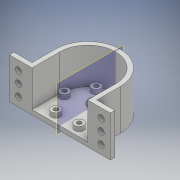
# Autodesk Inventor part: Mount for run motor
Saved by Autodesk Inventor 2018 (Build 220112000, 112)
## iProperties
Created: 2020-02-06
Part Number: Mount for run motor
Material: Типовые
Document SubType Name: Modeling
Designer: cosko
Density: 1 g/cm^3
Appearance: По умолчанию
Author: cosko
Autodesk Inventor part; units mm, degrees
ref_plane "YZ Plane" through (0, 0, 0) normal (1, 0, 0) x (0, 1, 0)
ref_plane "XZ Plane" through (0, 0, 0) normal (0, 1, 0) x (-1, 0, 0)
ref_plane "XY Plane" through (0, 0, 0) normal (0, 0, 1) x (1, 0, 0)
sketch "Эскиз1" plane through (0, 0, 0) normal (0, 0, 1) x (1, 0, 0)
  line L0 (0, 0) -> (0, 37) construction
  circle A0 centre (0, 18.5) radius 18.5 construction
  arc A1 (10.9545, 0) -> (-10.9545, 0) centre (0, 18.5) ccw construction
  line L1 (21.5, 18.5) -> (21.5, 0) construction
  line L2 (-21.5, 18.5) -> (-21.5, 0) construction
  line L3 (-21.5, 0) -> (21.5, 0) construction
  arc A2 (21.5, 18.5) -> (-21.5, 18.5) centre (0, 18.5) ccw construction
  arc A3 (21.5, 18.5) -> (-21.5, 18.5) centre (0, 18.5) ccw
  arc A4 (18.5, 18.5) -> (-18.5, 18.5) centre (0, 18.5) ccw
  line L4 (21.5, 0) -> (33.5, 0) construction
  line L5 (-21.5, 0) -> (-33.5, 0) construction
  line L6 (33.5, 0) -> (33.5, 3) construction
  line L7 (33.5, 3) -> (21.5, 3) construction
  line L8 (21.5, 3) -> (21.5, 18.5) construction
  line L9 (-33.5, 0) -> (-33.5, 3) construction
  line L10 (-33.5, 3) -> (-21.5, 3) construction
  line L11 (-21.5, 18.5) -> (-21.5, 3)
  line L12 (-21.5, 3) -> (-33.5, 3)
  line L13 (-33.5, 3) -> (-33.5, 0)
  line L14 (-33.5, 0) -> (-18.5, 0)
  line L15 (-18.5, 0) -> (-18.5, 18.5)
  line L16 (18.5, 18.5) -> (18.5, 0)
  line L17 (18.5, 0) -> (33.5, 0)
  line L18 (33.5, 0) -> (33.5, 3)
  line L19 (33.5, 3) -> (21.5, 3)
  line L20 (21.5, 3) -> (21.5, 18.5)
  dimension "d0" = 37
  dimension "d1" = 3
  dimension "d2" = 12
  dimension "d3" = 12
  dimension "d4" = 3
  dimension "d5" = 3
  constraints: 42 end point, 14 point on circle, 8 perpendicular, 7 point on line, 5 centre point, 5 tangent, 5 vertical, 3 horizontal, 1 collinear, 1 midpoint
  measures "d0" distance of L0.start L0.end
  measures "d1" radial gap between concentric circles of A0 A1
  measures "d2" distance of L1.end L4.end
  measures "d3" distance of L2.end L5.end
  measures "d4" distance of L4.end L6.end
  measures "d5" distance of L5.end L9.end
extrude "Выдавливание1" add sketch "Эскиз1" along normal blind 27
sketch "Эскиз2" plane through (0, 0, 0) normal (0, 0, -1) x (-1, 0, 0)
  arc A0 (21.5, 18.5) -> (-21.5, 18.5) centre (0, 18.5) ccw projected
  line L0 (-21.5, 3) -> (-21.5, 18.5) projected
  line L1 (-33.5, 3) -> (-21.5, 3) projected
  line L2 (-33.5, 0) -> (-33.5, 3) projected
  line L3 (-18.5, 0) -> (-33.5, 0) projected
  line L4 (-18.5, 18.5) -> (-18.5, 0) projected
  arc A1 (18.5, 18.5) -> (-18.5, 18.5) centre (0, 18.5) ccw projected
  line L5 (18.5, 0) -> (18.5, 18.5) projected
  line L6 (33.5, 0) -> (18.5, 0) projected
  line L7 (33.5, 3) -> (33.5, 0) projected
  line L8 (21.5, 3) -> (33.5, 3) projected
  line L9 (21.5, 18.5) -> (21.5, 3) projected
  circle A2 centre (0, 18.5) radius 18.5 construction
  circle A3 centre (0, 18.5) radius 15.5 construction
  circle A4 centre (-15.5, 18.5) radius 1.5
  circle A5 centre (-7.75, 5.0766) radius 1.5
  circle A6 centre (7.75, 5.0766) radius 1.5
  circle A7 centre (15.5, 18.5) radius 1.5
  circle A8 centre (7.75, 31.9234) radius 1.5
  circle A9 centre (-7.75, 31.9234) radius 1.5
  line L10 (0, 18.5) -> (0, 25.5) construction
  circle A10 centre (0, 25.5) radius 6
  line L11 (-18.5, 18.5) -> (-18.5, 0) projected
  line L12 (-18.5, 0) -> (18.5, 0)
  line L13 (18.5, 0) -> (18.5, 18.5) projected
  line L14 (18.5, 0) -> (18.5, 18.5)
  arc A11 (18.5, 18.5) -> (-18.5, 18.5) centre (0, 18.5) ccw
  line L15 (-18.5, 18.5) -> (-18.5, 0)
  point P0 (0, 0)
  dimension "d8" = 31
  dimension "d9" = 3
  dimension "d12" = 360
  dimension "d14" = 7
  dimension "d15" = 12
  constraints: 8 centre point, 8 end point, 3 coincident, 3 tangent, 2 perpendicular, 2 point on circle, 2 vertical, 1 collinear, 1 concentric, 1 horizontal alignment, 1 vertical alignment, 17 other
  measures "d9" diameter of A4
  measures "d14" distance of L10.start L10.end
  measures "d15" diameter of A10
extrude "Выдавливание2" add sketch "Эскиз2" against normal blind 3 contours L12 L4 A1 L5
sketch "Эскиз4" plane through (0, 0, 3) normal (0, 0, 1) x (1, 0, 0)
  circle A0 centre (0, 25.5) radius 6 projected
  circle A1 centre (7.75, 31.9234) radius 1.5 projected
  circle A2 centre (-7.75, 31.9234) radius 1.5 projected
  circle A3 centre (-15.5, 18.5) radius 1.5 projected
  circle A4 centre (-7.75, 5.0766) radius 1.5 projected
  circle A5 centre (7.75, 5.0766) radius 1.5 projected
  circle A6 centre (15.5, 18.5) radius 1.5 projected
  line L0 (-18.5, 0) -> (18.5, 0) projected
  line L1 (18.5, 18.5) -> (18.5, 0) projected
  arc A7 (18.5, 18.5) -> (-18.5, 18.5) centre (0, 18.5) ccw projected
  line L2 (-18.5, 0) -> (-18.5, 18.5) projected
  circle A8 centre (-7.75, 5.0766) radius 3
  circle A9 centre (-15.5, 18.5) radius 3
  circle A10 centre (-7.75, 31.9234) radius 3
  circle A11 centre (7.75, 31.9234) radius 3
  circle A12 centre (15.5, 18.5) radius 3
  circle A13 centre (7.75, 5.0766) radius 3
  point P0 (0, 0)
  dimension "d19" = 6
  dimension "d22" = 360
  constraints: 6 centre point, 3 coincident, 16 other
  measures "d19" diameter of A8
extrude "Выдавливание3" add sketch "Эскиз4" along normal blind 3 contours A12 | A11 | A10 | A9 | A8 | A13
sketch "Эскиз5" plane through (21.5, 3, 0) normal (0, 1, 0) x (1, 0, 0)
  line L0 (12, 0) -> (0, 0) projected
  line L1 (0, 0) -> (0, -27) projected
  line L2 (12, -27) -> (0, -27) projected
  line L3 (12, 0) -> (12, -27) projected
  line L4 (12, -27) -> (0, -27) construction
  line L5 (-3, -27) -> (12, -27) construction
  line L6 (6, -27) -> (6, 0) construction
  circle A0 centre (6, -13.5) radius 2
  circle A1 centre (6, -21) radius 2
  circle A2 centre (6, -6) radius 2
  circle A3 centre (6, -13.5) radius 2
  point P0 (-21.5, 0)
  dimension "d26" = 4
  dimension "d29" = 7.5
  dimension "d32" = 7.5
  constraints: 4 centre point, 4 end point, 3 midpoint, 2 vertical, 1 collinear, 6 other
  measures "d26" diameter of A0
  measures "d29" distance of A0.centre A1.centre
  measures "d32" distance of A0.centre A2.centre
extrude "Выдавливание4" cut sketch "Эскиз5" against normal blind 3 contours A0 | A1 | A2
ref_plane "РабПлоскость2" through (0, 3, 0) normal (-1, 0, 0) x (0, 0, 1)
mirror "Зеркальное отражение1" about plane through (0, 3, 0) normal (-1, 0, 0) of "Выдавливание4"
